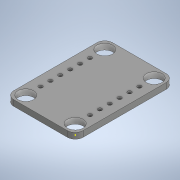
# Autodesk Inventor part: Adafruit_IMU
Saved by Autodesk Inventor 2020.3 (Build 243373000, 373)
## iProperties
Created: 2021-03-18
Part Number: Adafruit_IMU
Material: Ogólny
Document SubType Name: Modeling
Designer: patry
Density: 1 g/cm^3
Appearance: Domyślna
Author: patry
Autodesk Inventor part; units mm, degrees
ref_plane "YZ Plane" through (0, 0, 0) normal (1, 0, 0) x (0, 1, 0)
ref_plane "XZ Plane" through (0, 0, 0) normal (0, 1, 0) x (-1, 0, 0)
ref_plane "XY Plane" through (0, 0, 0) normal (0, 0, 1) x (1, 0, 0)
sketch "Szkic1" plane through (0, 0, 0) normal (0, 1, 0) x (-1, 0, 0)
  line L0 (2, 0) -> (15.8, 0)
  line L1 (17.8, -2) -> (17.8, -23.4)
  line L2 (15.8, -25.4) -> (2, -25.4)
  line L3 (0, -23.4) -> (0, -2)
  arc A0 (17.8, -2) -> (15.8, 0) centre (15.8, -2) ccw
  arc A1 (15.8, -25.4) -> (17.8, -23.4) centre (15.8, -23.4) ccw
  arc A2 (0, -23.4) -> (2, -25.4) centre (2, -23.4) ccw
  arc A3 (2, 0) -> (0, -2) centre (2, -2) ccw
  point P0 (0, 0)
  point P1 (17.8, -25.4)
  point P2 (17.8, 0)
  point P3 (0, -25.4)
  dimension "d0" = 17.8
  dimension "d1" = 25.4
  dimension "d2" = 2
  constraints: 8 end point, 8 point on circle, 8 point on line, 8 tangent, 4 centre point, 3 equal radius, 2 parallel, 1 horizontal, 1 perpendicular
  measures "d0" distance of point (17.8, -25.4) point (0, -25.4)
  measures "d1" distance of point (17.8, 0) point (17.8, -25.4)
  measures "d2" radius of A0
extrude "Wyciągnięcie proste1" add sketch "Szkic1" along normal blind 1.5
sketch "Szkic2" plane through (0, 1.5, 0) normal (0, 1, 0) x (1, 0, 0)
  line L0 (-2, 25.4) -> (-15.8, 25.4) projected
  line L1 (-17.8, 23.4) -> (-17.8, 2) projected
  line L2 (0, 2) -> (0, 23.4) projected
  point P0 (0, 0)
  point P1 (-2.54, 6.35)
  point P2 (-2.54, 8.89)
  point P3 (-2.54, 11.43)
  point P4 (-2.54, 13.97)
  point P5 (-15.26, 6.35)
  point P6 (-15.26, 8.89)
  point P7 (-15.26, 11.43)
  point P8 (-15.26, 13.97)
  point P9 (-15.26, 16.51)
  point P10 (-15.26, 19.05)
  point P11 (-2.54, 16.51)
  point P12 (-2.54, 19.05)
  dimension "d8" = 2.54
  dimension "d9" = 2.54
  dimension "d10" = 2.54
  dimension "d11" = 2.54
  dimension "d12" = 2.54
  dimension "d13" = 6.35
  dimension "d14" = 2.54
  dimension "d15" = 2.54
  dimension "d16" = 2.54
  dimension "d17" = 2.54
  dimension "d19" = 2.54
  constraints: 7 vertical alignment, 3 horizontal alignment
  measures "d8" distance of point (-15.26, 8.89) point (-15.26, 6.35)
  measures "d9" distance of point (-15.26, 11.43) point (-15.26, 8.89)
  measures "d10" distance of point (-15.26, 13.97) point (-15.26, 11.43)
  measures "d11" distance of point (-15.26, 16.51) point (-15.26, 13.97)
  measures "d12" distance of point (-15.26, 19.05) point (-15.26, 16.51)
  measures "d13" distance from line of L0 point (-15.26, 19.05)
  measures "d14" distance from line of L1 point (-15.26, 8.89)
  measures "d15" distance of point (-2.54, 11.43) point (-2.54, 13.97)
  measures "d16" distance of point (-2.54, 8.89) point (-2.54, 11.43)
  measures "d17" distance of point (-2.54, 6.35) point (-2.54, 8.89)
  measures "d19" distance from line of L2 point (-2.54, 13.97)
hole "Otwór1" at (-2.54, 1.5, -6.35) at (-2.54, 1.5, -8.89) at (-2.54, 1.5, -11.43) at (-2.54, 1.5, -13.97) at (-15.26, 1.5, -6.35) at (-15.26, 1.5, -8.89) at (-15.26, 1.5, -11.43) at (-15.26, 1.5, -13.97) at (-15.26, 1.5, -16.51) at (-15.26, 1.5, -19.05) at (-2.54, 1.5, -16.51) at (-2.54, 1.5, -19.05) direction (0, -1, 0) diameter 1 end through all
sketch "Szkic3" plane through (0, 1.5, 0) normal (0, 1, 0) x (1, 0, 0)
  point P0 (0, 0)
sketch "Szkic4" plane through (0, 1.5, 0) normal (0, 1, 0) x (1, 0, 0)
  circle A0 centre (-2.54, 13.97) radius 0.5 construction
  circle A1 centre (-2.54, 7.62) radius 0.5 construction
  line L0 (-2.54, 13.97) -> (-2.54, 7.62) construction
  line L1 (-2.54, 13.97) -> (-2.54, -5.3346) construction
  circle A2 centre (-2.54, 8.89) radius 0.5 construction
  line L2 (-2.54, 8.89) -> (-2.54, 22.9895) construction
  circle A3 centre (-2.54, 22.86) radius 2
  line L3 (-2, 25.4) -> (-15.8, 25.4) projected
  circle A4 centre (-2.54, 2.54) radius 2
  line L4 (-15.8, 0) -> (-2, 0) projected
  circle A5 centre (-15.26, 2.54) radius 2
  circle A6 centre (-15.26, 22.86) radius 2
  line L5 (-17.8, 23.4) -> (-17.8, 2) projected
  point P0 (0, 0)
  dimension "d27" = 4
  dimension "d28" = 2.54
  dimension "d29" = 4
  dimension "d30" = 2.54
  dimension "d33" = 4
  dimension "d34" = 4
  dimension "d35" = 2.54
  constraints: 6 end point, 4 centre point, 3 vertical, 2 point on line, 1 vertical alignment
  measures "d27" diameter of A3
  measures "d28" distance from line of L3 A3.centre
  measures "d29" diameter of A4
  measures "d30" distance from line of L4 A4.centre
  measures "d33" diameter of A5
  measures "d34" diameter of A6
  measures "d35" distance from line of L5 A5.centre
extrude "Wyciągnięcie proste2" cut sketch "Szkic4" against normal blind 10
equation "\"d8\" = d7"
equation "\"d9\" = d8"
equation "\"d10\" = d9"
equation "\"d11\" = d10"
equation "\"d12\" = d11"
equation "\"d13\" = 2.5 * d12"
equation "\"d14\" = d8"
equation "\"d16\" = d15"
equation "\"d17\" = d16"
equation "\"d6\" = d5"
equation "\"d7\" = d6"
equation "\"d5\" = 2.54"
